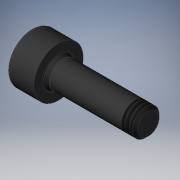
# Autodesk Inventor part: Slotted head cap screw ISO 4762 - M3x10
Saved by Autodesk Inventor 2019 (Build 230136000, 136)
## iProperties
Created: 2023-04-15
Part Number: Slotted head cap screw ISO 4762 - M3x10
Material: Generic
Catalog Web Link: www.cadenas.de
Description: ISO 4762-Hexagon socket head cap screw
Vendor: MISUMI
Document SubType Name: Modeling
Designer: psAdmin
Manufacturer: MISUMI
Mass: 0.13061 g
Surface Area: 2.04657 cm^2
Volume: 0.13061 cm^3
Density: 1 g/cm^3
Appearance: PSOLRGB-175-175-175
Category: PARTsolutions
Company: MISUMI
Title: Slotted head cap screw ISO 4762 - M3x10
Author: Cadenas PARTsolutions
Comments: Hexagon socket head cap screw
PSOL_IDENT_0: {$CADENAS_DATA/23d-libs/misumi/metric/accessories/din_en_iso_4762.prj},221 {VTYP=3D},{NB=Slotted hea
PSOL_IDENT_1: d cap screw ISO 4762 - M3x10},{LINA=Slotted head cap screw ISO 4762 - M3x10},{NN=ISO 4762},{DATE=13.
PSOL_IDENT_2: 07.2021 11:48:40},{GEOMDATE=21.06.2021 06:17:40},{VERSION=},{LINEID=310},{WBVAR=},{WBNUMERIC=}  {NB=
PSOL_IDENT_3: Zylinderschraube ISO 4762 - M3x10},{LINA=Zylinderschraube ISO 4762 - M3x10},{KT=DUMMY},{IDNR=},{D=3.
PSOL_IDENT_4: 000},{D3=2.387},{P=0.500},{L=10.000},{S=2.500},{HM=10.000},{DK=5.500},{DA=3.600},{DS=3.000},{E=2.870
PSOL_IDENT_5: },{K=3.000},{R=0.100},{T=1.300},{V=0.300},{DW=5.070},{W=1.150},{LF=0.510},{LG=1.500},{FORM=1.000},{N
PSOL_IDENT_6: ENN=M3x10}
NB: Slotted head cap screw ISO 4762 - M3x10
NN: ISO 4762
NT: Hexagon socket head cap screw
NBSYN: Slotted head cap screw ISO 4762 - $NENN.
LINA: Slotted head cap screw ISO 4762 - M3x10
CATALOG: Misumi
ROWDESC: M3x10
D: 3
D3: 2.387
P: 0.5
L: 10
S: 2.5
HM: 10
DK: 5.5
DA: 3.6
DS: 3
E: 2.87
K: 3
R: 0.1
T: 1.3
V: 0.3
DW: 5.07
W: 1.15
LF: 0.51
LG: 1.5
FORM: 1
SUPPLIER: MISUMI
ARTICLENO: Slotted head cap screw ISO 4762 - M3x10
BOMINFO: Slotted head cap screw ISO 4762 - M3x10
CREATOR: CADENAS GmbH
Autodesk Inventor part; units mm, degrees
sketch "Skizze_2" plane through (0, 0, 0) normal (0, 0, 1) x (1, 0, 0)
  line L0 (10, 0) -> (-0.4283, 0)
  line L1 (-0.4283, 0) -> (-1.15, 1.25)
  line L2 (-1.15, 1.25) -> (-3, 1.25)
  line L3 (-3, 1.25) -> (-3, 2.45)
  arc A0 (-2.7, 2.75) -> (-3, 2.45) centre (-2.7, 2.45) ccw
  line L4 (-2.7, 2.75) -> (0, 2.75)
  line L5 (0, 2.75) -> (0, 1.8)
  arc A1 (0, 1.8) -> (0.0562, 1.7101) centre (0.1, 1.8) ccw
  line L6 (0.0562, 1.7101) -> (0.4662, 1.5101)
  arc A2 (0.4662, 1.5101) -> (0.51, 1.5) centre (0.51, 1.6) ccw
  line L7 (0.51, 1.5) -> (9.6935, 1.5)
  line L8 (9.6935, 1.5) -> (10, 1.1935)
  line L9 (10, 1.1935) -> (10, 0)
  line L10 (10, 0) -> (-0.4283, 0)
  constraints: 22 end point, 6 point on circle, 3 centre point
revolve "Revolution1" add sketch "Skizze_2" angle 360 about axis through (10, 0, 0) along (1, 0, 0)
thread "Thread1" size "M3x0.5" class "6g" standard "ISO Metric profile" length 1.1935
sketch "Skizze_1" plane through (-1.15, 0, 0) normal (1, 0, 0) x (0, 0, -1)
  line L0 (-1.25, -0.7217) -> (0, -1.4434)
  line L1 (0, -1.4434) -> (1.25, -0.7217)
  line L2 (1.25, -0.7217) -> (1.25, 0.7217)
  line L3 (1.25, 0.7217) -> (0, 1.4434)
  line L4 (0, 1.4434) -> (-1.25, 0.7217)
  line L5 (-1.25, 0.7217) -> (-1.25, -0.7217)
  constraints: 12 end point
extrude "Extrusion1" cut sketch "Skizze_1" against normal blind 2.6
ref_plane "IP1_XY" through (0, 0, 0) normal (1, 0, 0) x (0, 0, -1)
ref_plane "IP1_YZ" through (0, 0, 0) normal (0, 0, -1) x (0, 1, 0)
ref_plane "IP1_ZX" through (0, 0, 0) normal (0, 1, 0) x (1, 0, 0)
ref_plane "IP2_XY" through (-3, 0, 0) normal (1, 0, 0) x (0, 0, -1)
ref_plane "IP2_YZ" through (-3, 0, 0) normal (0, 0, -1) x (0, 1, 0)
ref_plane "IP2_ZX" through (-3, 0, 0) normal (0, 1, 0) x (1, 0, 0)
ref_plane "IP3_XY" through (10, 0, 0) normal (1, 0, 0) x (0, 0, -1)
ref_plane "IP3_YZ" through (10, 0, 0) normal (0, 0, -1) x (0, 1, 0)
ref_plane "IP3_ZX" through (10, 0, 0) normal (0, 1, 0) x (1, 0, 0)
ref_plane "IP4_XY" through (0, 0, 0) normal (1, 0, 0) x (0, 0, -1)
ref_plane "IP4_YZ" through (0, 0, 0) normal (0, 0, -1) x (0, 1, 0)
ref_plane "IP4_ZX" through (0, 0, 0) normal (0, 1, 0) x (1, 0, 0)
body "Solid1"
